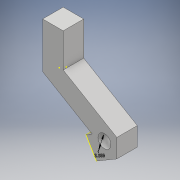
# Autodesk Inventor part: seeSaw
Saved by Autodesk Inventor 2018 (Build 220112000, 112)
## iProperties
Created: 2017-11-18
Part Number: seeSaw
Material: Generic
Document SubType Name: Modeling
Designer: Prakash
Density: 1 g/cm^3
Appearance: Default
Author: Prakash
Autodesk Inventor part; units mm, degrees
ref_plane "YZ Plane" through (0, 0, 0) normal (1, 0, 0) x (0, 1, 0)
ref_plane "XZ Plane" through (0, 0, 0) normal (0, 1, 0) x (-1, 0, 0)
ref_plane "XY Plane" through (0, 0, 0) normal (0, 0, 1) x (1, 0, 0)
sketch "Sketch1" plane through (0, 0, 0) normal (0, 1, 0) x (-1, 0, 0)
  line L0 (36.1277, -22.2455) -> (12, -36.4736)
  line L1 (12, -36.4736) -> (15.0796, -38.2896)
  line L2 (15.0796, -38.2896) -> (10, -46.9035)
  line L3 (10, -46.9035) -> (0, -41.0064)
  line L4 (36.1277, -22.2455) -> (36.1277, 0)
  line L5 (36.1277, 0) -> (26.1277, 0)
  line L6 (26.1277, 0) -> (26.1277, -16.5333)
  line L7 (26.1277, -16.5333) -> (0, -31.9408)
  line L8 (0, -31.9408) -> (0, -41.0064)
  line L9 (0, -36.4736) -> (12, -36.4736) construction
  circle A0 centre (6, -36.4736) radius 3.175
  point P0 (0, 0)
  dimension "d1" = 10
  dimension "d8" = 10
  dimension "d9" = 10
  dimension "d10" = 10
  dimension "d12" = 12
  dimension "d13" = 6.35
  dimension "d14" = 22.2455
  dimension "d17" = 61.056
  dimension "d19" = 28.0104
  constraints: 20 end point, 2 horizontal, 2 midpoint, 2 parallel, 2 point on line, 2 vertical, 1 centre point, 1 perpendicular
  measures "d1" distance between parallel lines of L4 L6
  measures "d8" distance between parallel lines of L7 L0
  measures "d9" distance between parallel lines of L3 L1
  measures "d10" horizontal distance of L3.end L2.end
  measures "d12" distance of L9.start L0.end
  measures "d13" diameter of A0
  measures "d14" distance of L0.start L4.end
  measures "d17" angle of L1 L0
  measures "d19" distance of L0.start L0.end
extrude "Extrusion1" add sketch "Sketch1" along normal blind 10
sketch "Sketch2" plane through (-15.0796, 0, -38.2896) normal (-0.8613822, 0, -0.5079575) x (-0.5079575, 0, 0.8613822)
  line L0 (0, 0) -> (-10, 0) projected
  line L1 (0, 0) -> (0, 10) projected
  line L2 (-10, 10) -> (0, 10) projected
  line L3 (-10, 0) -> (-10, 10) projected
  line L4 (-5, 10) -> (-5, 0) construction
  line L5 (-10, 5) -> (-5, 5) construction
  circle A0 centre (-5, 5) radius 2.5275
  circle A1 centre (-5, 5) radius 2.6545
  point P0 (25.3222, 0)
  dimension "d22" = 5.055
  dimension "d23" = 5.309
  constraints: 4 end point, 4 midpoint, 2 centre point, 2 coincident
  measures "d22" diameter of A0
  measures "d23" diameter of A1
extrude "Extrusion2" cut sketch "Sketch2" against normal blind 3.81 contours A0
sketch "Sketch3" plane through (-9.2579, 5, -40.6612) normal (-0.8613822, 0, -0.5079575) x (-0.5079575, 0, 0.8613822)
  line L0 (-5, 0) -> (0, 0) construction
  circle A0 centre (0, 0) radius 2.5275 projected
  circle A1 centre (0, 0) radius 2.5275
  point P0 (30.3222, -5)
  constraints: 1 centre point, 1 coincident, 1 concentric
body "Solid1"
